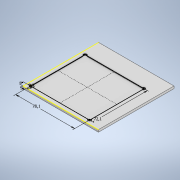
# Autodesk Inventor part: Part1
Saved by Autodesk Inventor 2022 (Build 260153000, 153)
## iProperties
Created: 2022-05-30
Part Number: Part1
Material: Generic
Document SubType Name: Modeling
Designer: atsel
Density: 1 g/cm^3
Appearance: Default
Author: atsel
Autodesk Inventor part; units mm, degrees
ref_plane "YZ Plane" through (0, 0, 0) normal (1, 0, 0) x (0, 1, 0)
ref_plane "XZ Plane" through (0, 0, 0) normal (0, 1, 0) x (-1, 0, 0)
ref_plane "XY Plane" through (0, 0, 0) normal (0, 0, 1) x (1, 0, 0)
sketch "Sketch1" plane through (0, 0, 0) normal (0, 1, 0) x (-1, 0, 0)
  line L0 (0, 0) -> (-100, 0)
  line L1 (-100, 0) -> (-100, -100)
  line L2 (-100, -100) -> (0, -100)
  line L3 (0, -100) -> (0, 0)
  dimension "d0" = 100
  dimension "d1" = 100
  constraints: 8 end point, 2 parallel, 1 horizontal, 1 perpendicular
  measures "d0" distance of L0.start L0.end
  measures "d1" distance of L0.end L1.end
extrude "Extrusion1" add sketch "Sketch1" along normal blind 3
sketch "Sketch2" plane through (0, 3, 0) normal (0, 1, 0) x (1, 0, 0)
  line L0 (5, 5) -> (83.1, 5)
  line L1 (83.1, 5) -> (83.1, 77.1)
  line L2 (83.1, 77.1) -> (5, 77.1)
  line L3 (5, 77.1) -> (5, 5)
  line L4 (0, 0) -> (100, 0) projected
  line L5 (0, 100) -> (0, 0) projected
  arc A0 (5, 7.4365) -> (7.4365, 5) centre (5.5, 5.5) ccw
  line L6 (44.05, 77.1) -> (44.05, 5) construction
  line L7 (5, 41.05) -> (83.1, 41.05) construction
  arc A1 (80.6635, 5) -> (83.1, 7.4365) centre (82.6, 5.5) ccw
  arc A2 (7.4365, 77.1) -> (5, 74.6635) centre (5.5, 76.6) ccw
  arc A3 (83.1, 74.6635) -> (80.6635, 77.1) centre (82.6, 76.6) ccw
  point P0 (80.6635, 5)
  point P1 (83.1, 7.4365)
  point P2 (83.1, 74.6635)
  point P3 (80.6635, 77.1)
  point P4 (7.4365, 77.1)
  point P5 (5, 74.6635)
  dimension "d4" = 78.1
  dimension "d5" = 72.1
  dimension "d6" = 5
  dimension "d7" = 5
  dimension "d10" = 0.5
  dimension "d11" = 0.5
  dimension "d12" = 2
  constraints: 12 end point, 9 symmetric about line, 8 point on circle, 4 centre point, 4 midpoint, 2 parallel, 2 point on line, 1 horizontal, 1 perpendicular, 3 other
  measures "d4" distance of L0.start L0.end
  measures "d5" distance of L0.end L1.end
  measures "d6" distance between parallel lines of L4 L0
  measures "d7" distance between parallel lines of L5 L3
  measures "d10" distance from line of L3 A0.centre
  measures "d11" distance from line of L0 A0.centre
  measures "d12" radius of A0
extrude "Extrusion2" cut sketch "Sketch2" against normal blind 1
fillet "Fillet1" radius 1 8 edges at (5, 2.5, -7.4365) (7.4365, 2.5, -5) (83.1, 2.5, -7.4365) (80.6635, 2.5, -5) (83.1, 2.5, -74.6635) (80.6635, 2.5, -77.1) (7.4365, 2.5, -77.1) (5, 2.5, -74.6635)
body "Solid1"
